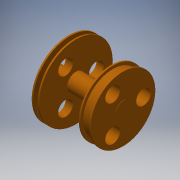
# Autodesk Inventor part: PulleyMotor
Saved by Autodesk Inventor 2019 (Build 230136000, 136)
## iProperties
Created: 2017-01-18
Part Number: PulleyMotor
Document SubType Name: Modeling
Designer: Administrator
Density: 1 g/cm^3
Mass: 2.43589 g
Surface Area: 27.7969 cm^2
Volume: 2.43589 cm^3
Material: Generic
Appearance: Orange
Author: Administrator
Autodesk Inventor part; units mm, degrees
ref_plane "YZ Plane" through (0, 0, 0) normal (1, 0, 0) x (0, 1, 0)
ref_plane "XZ Plane" through (0, 0, 0) normal (0, 1, 0) x (-1, 0, 0)
ref_plane "XY Plane" through (0, 0, 0) normal (0, 0, 1) x (1, 0, 0)
sketch "Sketch1" plane through (0, 0, 0) normal (0, 0, 1) x (1, 0, 0)
  line L0 (0, 0) -> (0, 3)
  line L1 (0, 3) -> (12, 3)
  line L2 (12, 3) -> (12, 11)
  line L3 (12, 11) -> (12.5, 11)
  line L4 (12.5, 11) -> (12.5, 10)
  line L5 (12.5, 10) -> (15.5, 10)
  line L6 (15.5, 10) -> (15.5, 11)
  line L7 (15.5, 11) -> (16, 11)
  line L8 (16, 11) -> (16, 0)
  line L9 (16, 0) -> (0, 0)
  dimension "d0" = 3
  dimension "d1" = 12
  dimension "d2" = 0.5
  dimension "d3" = 10
  dimension "d4" = 0.5
  dimension "d5" = 1
  dimension "d6" = 3
  constraints: 20 end point, 9 parallel, 1 perpendicular, 1 vertical, 1 other
  measures "d0" distance between parallel lines of L1 L9
  measures "d1" distance between parallel lines of L0 L2
  measures "d2" distance of L2.end L3.end
  measures "d3" distance between parallel lines of L5 L9
  measures "d4" distance of L6.end L7.end
  measures "d5" distance between parallel lines of L3 L5
  measures "d6" distance of L4.end L5.end
revolve "Revolution1" add sketch "Sketch1" angle 360 about axis through (16, 0, 0) along (-1, 0, 0)
sketch "Sketch2" plane through (0, 0, 0) normal (0, 0, 1) x (1, 0, 0)
  line L0 (0, -3) -> (0, 3) projected
  line L1 (0, 0) -> (-2.5, 0)
  line L2 (-2.5, 0) -> (-2.5, 12.5)
  line L3 (-2.5, 12.5) -> (0, 12.5) construction
  line L4 (0, 12.5) -> (0, 0)
  line L5 (-1.25, 12.5) -> (-1.25, 11) construction
  line L6 (-1.25, 11) -> (-1.5981, 11)
  line L7 (-1.5981, 11) -> (-2, 12.5)
  line L8 (-0.9019, 11) -> (-0.5, 12.5)
  line L9 (-0.9019, 11) -> (-1.25, 11)
  line L10 (-2, 12.5) -> (-2.5, 12.5)
  line L11 (-0.5, 12.5) -> (0, 12.5)
  dimension "d8" = 12.5
  dimension "d9" = 2.5
  dimension "d10" = 1.5
  dimension "d11" = 15
  dimension "d12" = 0.75
  constraints: 22 end point, 4 collinear, 3 perpendicular, 2 midpoint, 2 parallel, 2 symmetric about line, 1 point on line
  measures "d8" distance between parallel lines of L3 L1
  measures "d9" distance between parallel lines of L2 L4
  measures "d10" distance of L5.start L5.end
  measures "d11" angle of L7 L5
  measures "d12" distance from line of L5 L7.end
revolve "Revolution2" add sketch "Sketch2" angle 360 about axis through (0, 0, 0) along (-1, 0, 0)
sketch "Sketch3" plane through (-2.5, 0, 0) normal (-1, 0, 0) x (0, 0, 1)
  circle A0 centre (0, 0) radius 12.5 projected
  circle A1 centre (0, 0) radius 2
  dimension "d14" = 4
  constraints: 1 centre point, 1 coincident
  measures "d14" diameter of A1
extrude "Extrusion1" add sketch "Sketch3" along normal blind 4 contours A1
sketch "Sketch4" plane through (16, 0, 0) normal (1, 0, 0) x (0, 0, -1)
  circle A0 centre (0, 0) radius 10.5
  circle A1 centre (0, 0) radius 10
  circle A2 centre (0, 0) radius 11
  circle A3 centre (0, 7) radius 2.5
  circle A4 centre (0, 0) radius 3 construction
  dimension "d17" = 7
  dimension "d18" = 5
  dimension "d19" = 6
  constraints: 5 centre point, 1 coincident
  measures "d17" distance of A3.centre A0.centre
  measures "d18" diameter of A3
  measures "d19" diameter of A4
extrude "Extrusion2" cut sketch "Sketch4" against normal through all contours A3
pattern_circular "Circular Pattern1" count 3 over 360 about axis through (6, 0, 0) along (1, 0, 0) of "Extrusion2"
sketch "Sketch5" plane through (16, 0, 0) normal (1, 0, 0) x (0, 0, -1)
  circle A0 centre (0, 0) radius 11 projected
  circle A1 centre (0, 0) radius 2.5
  dimension "d25" = 5
  constraints: 1 centre point, 1 coincident
  measures "d25" diameter of A1
extrude "Extrusion3" add sketch "Sketch5" along normal blind 0.1 contours A1
body "Solid1"
